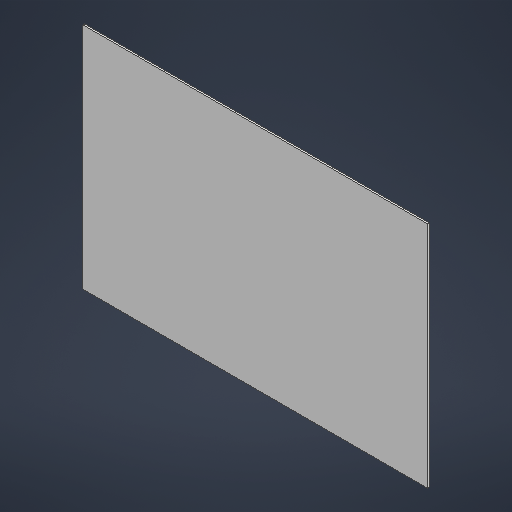
# Autodesk Inventor part: parte trasera
Saved by Autodesk Inventor 2027 (Build 310192060, 192F)
## iProperties
Created: 2026-09-04
Part Number: parte trasera
Material: Genérico
Document SubType Name: Modeling
Designer: Leandro
Density: 1 g/cm^3
Appearance: Valor por defecto
Author: Leandro
Autodesk Inventor part; units mm, degrees
ref_plane "YZ Plane" through (0, 0, 0) normal (1, 0, 0) x (0, 1, 0)
ref_plane "XZ Plane" through (0, 0, 0) normal (0, 1, 0) x (-1, 0, 0)
ref_plane "XY Plane" through (0, 0, 0) normal (0, 0, 1) x (1, 0, 0)
sketch "Boceto1" plane through (0, 0, 0) normal (0, 0, 1) x (1, 0, 0)
  line L0 (52.3312, 188.1492) -> (353.3312, 188.1492)
  line L1 (353.3312, 188.1492) -> (353.3312, -11.8508)
  line L2 (353.3312, -11.8508) -> (52.3312, -11.8508)
  line L3 (52.3312, -11.8508) -> (52.3312, 188.1492)
  point P0 (0, 0)
  dimension "d0" = 301
  dimension "d1" = 200
  constraints: 8 end point, 2 parallel, 1 horizontal, 1 perpendicular
  measures "d0" distance of L1.end L2.end
  measures "d1" distance of L0.end L1.end
extrude "Extrusión1" add sketch "Boceto1" along normal mid plane 1.5
